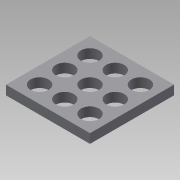
# Autodesk Inventor part: OlloGrid
Saved by Autodesk Inventor 2014 (Build 180170000, 170)
## iProperties
Created: 2014-03-04
Part Number: OlloGrid
Material: Générique
Document SubType Name: Modeling
Designer: Grégoire
Density: 1 g/cm^3
Appearance: Par défaut
Author: Grégoire
Autodesk Inventor part; units mm, degrees
ref_plane "YZ Plane" through (0, 0, 0) normal (1, 0, 0) x (0, 1, 0)
ref_plane "XZ Plane" through (0, 0, 0) normal (0, 1, 0) x (-1, 0, 0)
ref_plane "XY Plane" through (0, 0, 0) normal (0, 0, 1) x (1, 0, 0)
sketch "OlloGrid" plane through (0, 0, 0) normal (0, 0, 1) x (1, 0, 0)
  line L0 (0, 0) -> (20, 0)
  line L1 (20, 0) -> (20, 20)
  line L2 (20, 20) -> (0, 20)
  line L3 (0, 20) -> (0, 0)
  circle A0 centre (4, 16) radius 2.15
  line L4 (4, 16) -> (4, 20) construction
  line L5 (4, 16) -> (0, 16) construction
  circle A1 centre (10, 16) radius 2.15
  circle A2 centre (16, 16) radius 2.15
  circle A3 centre (4, 10) radius 2.15
  circle A4 centre (10, 10) radius 2.15
  circle A5 centre (16, 10) radius 2.15
  circle A6 centre (4, 4) radius 2.15
  circle A7 centre (10, 4) radius 2.15
  circle A8 centre (16, 4) radius 2.15
  dimension "d0" = 20
  dimension "d4" = 4.3
  dimension "d5" = 4
  dimension "d8" = 6
  dimension "d11" = 6
  constraints: 12 end point, 9 centre point, 5 perpendicular, 2 horizontal, 2 parallel, 2 point on line, 1 vertical, 16 other
  measures "d0" distance of L2.end L0.start
  measures "d4" diameter of A0
  measures "d5" distance of L4.start L5.end
  measures "d8" distance of L4.start A1.centre
  measures "d11" distance of L4.start A3.centre
extrude "Ollo" add sketch "OlloGrid" along normal blind 2.2
